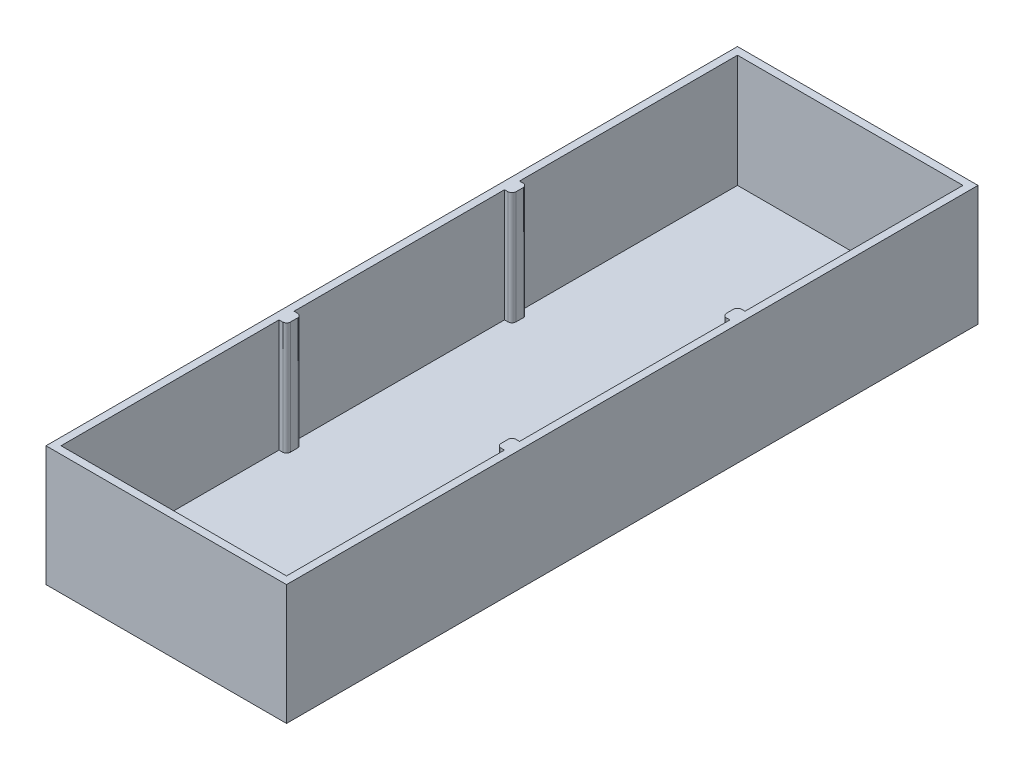
# Autodesk Inventor part: lab
Saved by Autodesk Inventor 2020 (Build 240168000, 168)
## iProperties
Created: 2022-09-26
Part Number: lab
Material: Типовые
Document SubType Name: Modeling
Designer: akapu
Density: 1 g/cm^3
Appearance: По умолчанию
Author: akapu
Autodesk Inventor part; units mm, degrees
ref_plane "YZ Plane" through (0, 0, 0) normal (1, 0, 0) x (0, 1, 0)
ref_plane "XZ Plane" through (0, 0, 0) normal (0, 1, 0) x (-1, 0, 0)
ref_plane "XY Plane" through (0, 0, 0) normal (0, 0, 1) x (1, 0, 0)
sketch "Эскиз1" plane through (0, 0, 0) normal (0, 1, 0) x (-1, 0, 0)
  line L0 (0, 0) -> (-300, 0)
  line L1 (-300, 0) -> (-300, -900)
  line L2 (-300, -900) -> (0, -900)
  line L3 (0, -900) -> (0, 0)
  line L4 (-300, 0) -> (0, 0)
  line L5 (0, 0) -> (0, -300)
  line L6 (0, -300) -> (-300, -300)
  line L7 (-300, -300) -> (-300, 0)
  line L8 (0, -900) -> (-300, -900)
  line L9 (-300, -900) -> (-300, -600)
  line L10 (-300, -600) -> (0, -600)
  line L11 (0, -600) -> (0, -900)
  dimension "d0" = 300
  dimension "d1" = 900
  constraints: 24 end point, 6 parallel, 3 horizontal, 3 perpendicular
  measures "d0" distance of L2.end L1.end
  measures "d1" distance of L1.end L0.end
extrude "Выдавливание1" add sketch "Эскиз1" along normal blind 10
sketch "Эскиз2" plane through (0, 0, 0) normal (0, -1, 0) x (1, 0, 0)
  line L0 (0, -900) -> (0, 0) projected
  line L1 (0, 0) -> (-10, 0)
  line L2 (-10, 0) -> (-10, -900)
  line L3 (-10, -900) -> (0, -900)
  line L4 (0, -900) -> (0, 0)
  line L5 (0, 0) -> (300, 0) projected
  line L6 (300, 0) -> (310, 0)
  line L7 (310, 0) -> (310, -900)
  line L8 (310, -900) -> (300, -900)
  line L9 (300, -900) -> (300, 0)
  line L10 (-10, -900) -> (310, -900)
  line L11 (310, -900) -> (310, -910)
  line L12 (310, -910) -> (-10, -910)
  line L13 (-10, -910) -> (-10, -900)
  line L14 (-10, 0) -> (310, 0)
  line L15 (310, 0) -> (310, 10)
  line L16 (310, 10) -> (-10, 10)
  line L17 (-10, 10) -> (-10, 0)
  dimension "d8" = 10
  dimension "d9" = 10
  dimension "d10" = 10
  dimension "d11" = 10
  constraints: 32 end point, 8 parallel, 4 horizontal, 4 perpendicular, 2 point on line
  measures "d8" distance of L3.end L2.end
  measures "d9" distance of L7.end L8.end
  measures "d10" distance of L10.end L11.end
  measures "d11" distance of L15.end L14.end
extrude "Выдавливание2" add sketch "Эскиз2" against normal blind 160 contours L3 L2 L1 L0 | L10 L8 L11 L12 L13 L3 | L1 L17 L16 L15 L6 L5 | L9 L6 L7 L8
ref_plane "РабПлоскость2" through (150, 0, 10) normal (1, 0, 0) x (0, 0, -1)
ref_plane "РабПлоскость3" through (-10, 0, -450) normal (0, 0, 1) x (1, 0, 0)
sketch "Эскиз3" plane through (0, 10, 0) normal (0, 1, 0) x (1, 0, 0)
  line L0 (300, 0) -> (0, 0) projected
  line L1 (300, 0) -> (300, 300)
  line L2 (300, 900) -> (300, 0) projected
  line L3 (300, 300) -> (300, 600)
  line L4 (310, -10) -> (310, 910) projected
  line L5 (290, 610) -> (310, 610)
  line L6 (310, 610) -> (310, 590)
  line L7 (310, 590) -> (290, 590)
  line L8 (290, 590) -> (290, 610)
  line L9 (290, 610) -> (310, 590) construction
  line L10 (310, 610) -> (290, 590) construction
  line L11 (290, 310) -> (310, 310)
  line L12 (310, 310) -> (310, 290)
  line L13 (310, 290) -> (290, 290)
  line L14 (290, 290) -> (290, 310)
  line L15 (290, 310) -> (310, 290) construction
  line L16 (310, 310) -> (290, 290) construction
  line L17 (10, 610) -> (-10, 610)
  line L18 (-10, 610) -> (-10, 590)
  line L19 (-10, 590) -> (10, 590)
  line L20 (10, 590) -> (10, 610)
  line L21 (0, 0) -> (0, 900) projected
  line L22 (10, 610) -> (-10, 590) construction
  line L23 (-10, 610) -> (10, 590) construction
  line L24 (-10, 910) -> (-10, -10) projected
  line L25 (10, 310) -> (-10, 310)
  line L26 (-10, 310) -> (-10, 290)
  line L27 (-10, 290) -> (10, 290)
  line L28 (10, 290) -> (10, 310)
  line L29 (10, 310) -> (-10, 290) construction
  line L30 (-10, 310) -> (10, 290) construction
  point P0 (0, 600)
  point P1 (0, 300)
  point P2 (0, 310)
  point P3 (0, 590)
  point P4 (300, 590)
  point P5 (300, 310)
  dimension "d14" = 300
  dimension "d15" = 300
  dimension "d16" = 20
  dimension "d17" = 20
  constraints: 52 end point, 10 point on line, 8 midpoint, 8 parallel, 4 horizontal, 4 perpendicular
  measures "d14" distance of L0.start L1.end
  measures "d15" distance of L1.end L3.end
  measures "d16" distance of L5.end L6.end
  measures "d17" distance of L11.end L12.end
extrude "Выдавливание3" add sketch "Эскиз3" along normal blind 150
fillet "Сопряжение1" radius 5 8 edges at (290, 85, -610) (290, 85, -590) (290, 85, -310) (290, 85, -290) (10, 85, -310) (10, 85, -290) (10, 85, -610) (10, 85, -590)
